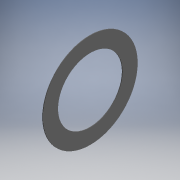
# Autodesk Inventor part: 607ZZ Shield
Saved by Autodesk Inventor 2017.3 (Build 213256000, 256)
## iProperties
Part Number: 607ZZ Shield
Material: Generic
Catalog Web Link: www.cadenas.de
Description: Six types s-Metric system sizes
Vendor: NTN
Document SubType Name: Modeling
Designer: partserver
Manufacturer: NTN
Mass: 0.0109107 g
Surface Area: 2.22513 cm^2
Volume: 0.0109107 cm^3
Density: 1 g/cm^3
Appearance: PSOLRGB-128-128-128
Category: PARTsolutions
Company: NTN
Title: 607ZZ Shield
Author: Cadenas PARTsolutions
Comments: Metric system sizes
PSOL_IDENT_0: {$CADENAS_DATA\23d-libs\ntn\ball_roller_bearings\miniature_extra_small_bb\metric_system_sizes\mss_s.
PSOL_IDENT_1: prj},172 {VTYP=3D},{NB=607ZZ Shield},{LINA=607ZZ Shield},{NN=Six types s},{DATE=21.12.2021 04:23:05}
PSOL_IDENT_2: ,{GEOMDATE=06.03.2020 10:08:02},{VERSION=},{LINEID=12950},{WBVAR=},{WBNUMERIC=}  {NB=607ZZ Shield},{
PSOL_IDENT_3: LINA=607ZZ Shield},{KT=DUMMY},{IDNR=},{SD=7.0},{D=19},{B=6.0},{R=0.30},{ORDER=607ZZ},{CR=2 240},{COR=
PSOL_IDENT_4: 910},{CRF=228},{CORF=93},{LSG=34 000},{LSO=40 000},{MASS=8.00},{ORDER1=607},{D1=0.0},{D2=0.0},{C1=0.
PSOL_IDENT_5: 0},{C2=0.0},{WSS=607ZZ},{WDS=ZZ},{UTWF=0},{FORSS=0},{FORDS=0},{DA1=9},{DA2=10,4},{DA=17},{RAS=0,3},{
PSOL_IDENT_6: MASS1=0.00},{B1=6.0},{VERS=3},{X=6},{N=7},{O=40.82},{RB=1.776}
NB: 607ZZ Shield
NN: Six types s
NT: Metric system sizes
NBSYN: $ORDER. Shield
LINA: 607ZZ Shield
CATALOG: NTN Corporation
SD: 7
D: 19
B: 6
R: 0.3
CR: 2 240
COR: 910
CRF: 228
CORF: 93
LSG: 34 000
LSO: 40 000
MASS: 8
ORDER1: 607
D1: 0
D2: 0
C1: 0
C2: 0
WSS: 607ZZ
WDS: ZZ
UTWF: 0
FORSS: 0
FORDS: 0
DA1: 9
DA2: 10,4
DA: 17
RAS: 0,3
MASS1: 0
B1: 6
VERS: 3
SUPPLIER: NTN
ARTICLENO: 607ZZ Shield
BOMINFO: 607ZZ Shield
CREATOR: CADENAS GmbH
Autodesk Inventor part; units mm, degrees
sketch "Sketch_1" plane through (0, 0, 0) normal (0, 0, 1) x (1, 0, 0)
  line L0 (-0.033, 0) -> (-0.135, 0)
  line L1 (-0.135, 7.964) -> (-0.135, 5.42)
  line L2 (-0.135, 5.42) -> (-0.033, 5.42)
  line L3 (-0.033, 5.42) -> (-0.033, 7.964)
  line L4 (-0.033, 7.964) -> (-0.135, 7.964)
  constraints: 10 end point
revolve "Revolution1" add sketch "Sketch_1" angle 360 about axis through (-0.033, 0, 0) along (1, 0, 0)
ref_plane "mss_s_XY" through (0, 0, 0) normal (1, 0, 0) x (0, 0, -1)
ref_plane "mss_s_YZ" through (0, 0, 0) normal (0, 0, -1) x (0, 1, 0)
ref_plane "mss_s_ZX" through (0, 0, 0) normal (0, 1, 0) x (1, 0, 0)
body "Solid1"
